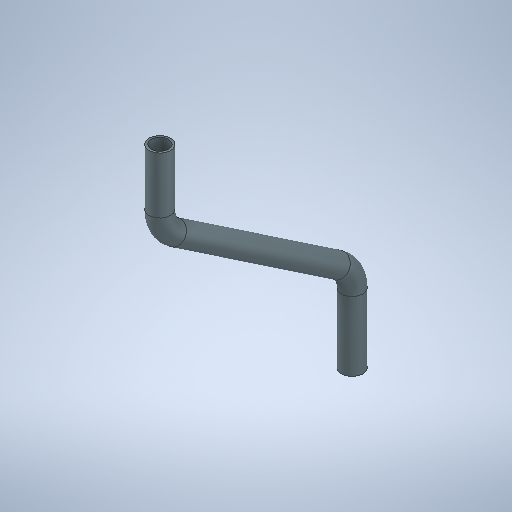
# Autodesk Inventor part: 158
Saved by Autodesk Inventor 2025.1 (Build 291241000, 241)
## iProperties
Created: 2024-08-03
Part Number: 158
Material: Iron, Gray
Document SubType Name: Modeling
Designer: ffogue
Density: 7.15 g/cm^3
Appearance: Lead
Author: ffogue
Autodesk Inventor part; units mm, degrees
ref_plane "YZ Plane" through (0, 0, 0) normal (1, 0, 0) x (0, 1, 0)
ref_plane "XZ Plane" through (0, 0, 0) normal (0, 1, 0) x (-1, 0, 0)
ref_plane "XY Plane" through (0, 0, 0) normal (0, 0, 1) x (1, 0, 0)
sketch "Sketch1" plane through (0, 0, 0) normal (0, 0, 1) x (1, 0, 0)
  circle A0 centre (0, 0) radius 2.5
  dimension "d0" = 5
  constraints: 1 centre point, 1 coincident
  measures "d0" diameter of A0
sketch "Sketch3" plane through (0, 0, 0) normal (1, 0, 0) x (0, 1, 0)
  line L0 (0, 0) -> (0, -13.011)
  line L1 (3.3076, -19.2298) -> (41.1924, -44.7702)
  line L2 (44.5, -50.989) -> (44.5, -67)
  arc A0 (0, -13.011) -> (3.3076, -19.2298) centre (7.5, -13.011) ccw
  arc A1 (44.5, -50.989) -> (41.1924, -44.7702) centre (37, -50.989) ccw
  point P0 (0, -17)
  point P1 (44.5, -47)
  dimension "d1" = 17
  dimension "d2" = 30
  dimension "d3" = 44.5
  dimension "d4" = 20
  dimension "d5" = 7.5
  constraints: 6 end point, 4 point on circle, 4 point on line, 4 tangent, 2 centre point, 1 equal radius, 1 parallel, 1 vertical
  measures "d1" distance of point (0, -17) L0.start
  measures "d2" vertical distance of point (44.5, -47) point (0, -17)
  measures "d3" distance from line of L0.start L2
  measures "d4" distance of point (44.5, -47) L2.end
  measures "d5" radius of A0
sweep "Sweep1" add profiles "Sketch1" path "Sketch3"
shell "Shell1" thickness 0.5 removed faces 2 at (1.2757, -0.3919, 0) at (0.6238, 43.9474, -67)
body "Solid1"
